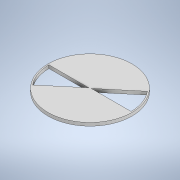
# Autodesk Inventor part: Деталь4
Saved by Autodesk Inventor 2022 (Build 260153000, 153)
## iProperties
Created: 2023-03-15
Part Number: Деталь4
Material: Типовые
Document SubType Name: Modeling
Designer: lrnto01
Density: 1 g/cm^3
Appearance: По умолчанию
Author: lrnto01
Autodesk Inventor part; units mm, degrees
ref_plane "YZ Plane" through (0, 0, 0) normal (1, 0, 0) x (0, 1, 0)
ref_plane "XZ Plane" through (0, 0, 0) normal (0, 1, 0) x (-1, 0, 0)
ref_plane "XY Plane" through (0, 0, 0) normal (0, 0, 1) x (1, 0, 0)
sketch "Эскиз1" plane through (0, 0, 0) normal (0, 1, 0) x (-1, 0, 0)
  circle A0 centre (0, 0) radius 65
  line L0 (0.182, -0.5) -> (62.998, -0.5)
  line L1 (62.998, 0.5) -> (1.3737, 0.5)
  line L2 (1.3737, 0.5) -> (48.5807, 40.1113)
  line L3 (47.9379, 40.8774) -> (-0.182, 0.5)
  line L4 (-0.182, 0.5) -> (-62.998, 0.5)
  line L5 (-62.998, -0.5) -> (-1.3737, -0.5)
  line L6 (-1.3737, -0.5) -> (-48.5807, -40.1113)
  line L7 (-47.9379, -40.8774) -> (0.182, -0.5)
  arc A1 (-62.998, -0.5) -> (-48.5807, -40.1113) centre (0, 0) ccw
  arc A2 (47.9379, 40.8774) -> (-62.998, 0.5) centre (0, 0) ccw
  arc A3 (-47.9379, -40.8774) -> (62.998, -0.5) centre (0, 0) ccw
  arc A4 (62.998, 0.5) -> (48.5807, 40.1113) centre (0, 0) ccw
  dimension "d1" = 130
  constraints: 16 end point, 8 point on circle, 5 centre point, 2 coincident, 1 horizontal
  measures "d1" diameter of A0
extrude "Выдавливание1" add sketch "Эскиз1" along normal blind 5 contours A0 | L0 A3 L7 | L3 L4 A2
